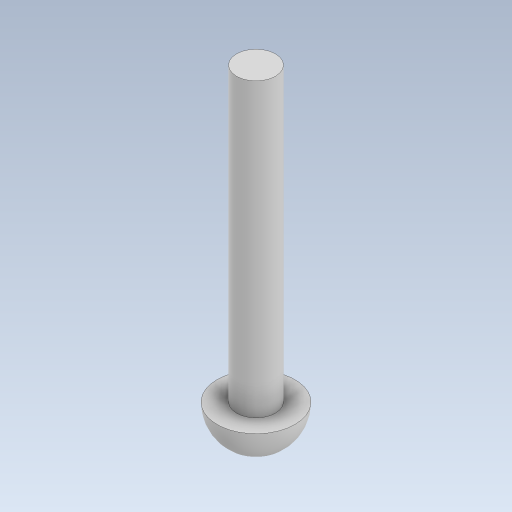
# Autodesk Inventor part: screw_4_12
Saved by Autodesk Inventor 2023 (Build 270158000, 158)
## iProperties
Created: 2023-05-16
Part Number: screw_4_12
Material: 一般
Document SubType Name: Modeling
Designer: Johnny Jou
Density: 1 g/cm^3
Appearance: 預設
Author: Johnny Jou
Autodesk Inventor part; units mm, degrees
ref_plane "YZ Plane" through (0, 0, 0) normal (1, 0, 0) x (0, 1, 0)
ref_plane "XZ Plane" through (0, 0, 0) normal (0, 1, 0) x (-1, 0, 0)
ref_plane "XY Plane" through (0, 0, 0) normal (0, 0, 1) x (1, 0, 0)
sketch "草圖2" plane through (0, 0, 0) normal (0, 0, 1) x (1, 0, 0)
  line L0 (0, -11.7941) -> (0, 36.9657) projected
  line L1 (0, 30) -> (-2, 30)
  line L2 (-2, 30) -> (-2, 0)
  line L3 (-2, 0) -> (0, 0)
  line L4 (0, 0) -> (0, 30)
  line L5 (-2, 0) -> (-4, 0)
  arc A0 (-4, 0) -> (0, -4) centre (0, 0) ccw
  dimension "d6" = 30
  dimension "d7" = 2
  dimension "d8" = 2
  constraints: 10 end point, 2 horizontal, 2 parallel, 2 point on circle, 2 point on line, 1 centre point, 1 coincident, 1 perpendicular
  measures "d6" distance of L1.end L2.end
  measures "d7" distance of L1.start L1.end
  measures "d8" distance of L2.end L5.end
revolve "迴轉1" add sketch "草圖2" angle 360 about axis through (0, -10, 0) along (0, 1, 0)
